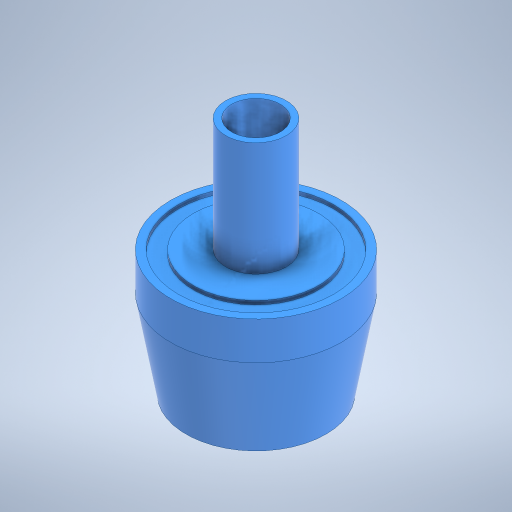
# Autodesk Inventor part: FlangeCone
Saved by Autodesk Inventor 2024 (Build 280153000, 153)
## iProperties
Created: 2023-09-22
Part Number: FlangeCone
Material: Brass
Document SubType Name: Modeling
Designer: schanen
Density: 8.49 g/cm^3
Appearance: Cyan
Author: schanen
Autodesk Inventor part; units mm, degrees
ref_plane "YZ Plane" through (0, 0, 0) normal (1, 0, 0) x (0, 1, 0)
ref_plane "XZ Plane" through (0, 0, 0) normal (0, 1, 0) x (-1, 0, 0)
ref_plane "XY Plane" through (0, 0, 0) normal (0, 0, 1) x (1, 0, 0)
sketch "Sketch1" plane through (0, 0, 0) normal (0, 0, 1) x (1, 0, 0)
  line L0 (-6.4, 63) -> (-6.4, 48)
  line L1 (-6.4, 48) -> (-6.1, 48)
  line L2 (-6.1, 48) -> (-6.1, 23)
  line L3 (-6.1, 23) -> (-17.5, 23)
  line L4 (-17.5, 23) -> (-17.5, 0)
  line L5 (-17.5, 0) -> (-18.4445, 0)
  line L6 (-18.4445, 0) -> (-22.5, 23)
  line L7 (-22.5, 23) -> (-22.5, 33)
  line L8 (-22.5, 33) -> (-20.5, 33)
  line L9 (-20.5, 33) -> (-20.5, 32)
  line L10 (-20.5, 32) -> (-16.5, 32)
  line L11 (-16.5, 32) -> (-16.5, 33)
  line L12 (-16.5, 33) -> (-8, 33)
  line L13 (-8, 33) -> (-8, 63)
  line L14 (-8, 63) -> (-6.4, 63)
  line L15 (0, -12.6) -> (0, 75.6) projected
  point P0 (0, 0)
  point P1 (-17.9722, 0)
  dimension "d0" = 23
  dimension "d1" = 15
  dimension "d2" = 30
  dimension "d3" = 10
  dimension "d4" = 17.5
  dimension "d5" = 6.1
  dimension "d6" = 6.4
  dimension "d7" = 8
  dimension "d8" = 22.5
  dimension "d9" = 10
  dimension "d10" = 4
  dimension "d11" = 20.5
  dimension "d12" = 1
  constraints: 30 end point, 11 perpendicular, 3 point on line, 1 horizontal alignment, 1 midpoint, 1 parallel, 1 vertical
  measures "d0" distance of L3.end L4.end
  measures "d1" distance of L0.start L0.end
  measures "d2" distance of L12.end L13.end
  measures "d3" distance of L6.end L7.end
  measures "d4" distance from line of point (0, 0) L4
  measures "d5" distance from line of point (0, 0) L2
  measures "d6" distance from line of point (0, 0) L0
  measures "d7" distance from line of point (0, 0) L13
  measures "d8" distance from line of point (0, 0) L7
  measures "d9" angle of L7 L6
  measures "d10" distance between parallel lines of L9 L11
  measures "d11" distance from line of point (0, 0) L9
  measures "d12" distance between parallel lines of L12 L10
revolve "Revolution1" add sketch "Sketch1" angle 360 about axis through (0, -10, 0) along (0, 1, 0)
sketch "Sketch2" plane through (0, 23, 0) normal (0, -1, 0) x (1, 0, 0)
  circle A0 centre (0, 0) radius 11 construction
  point P0 (0, 11)
  point P1 (-9.5263, -5.5)
  point P2 (9.5263, -5.5)
  dimension "d14" = 22
  dimension "d15" = 120
  dimension "d16" = 120
  constraints: 3 point on circle, 1 centre point, 1 coincident
  measures "d14" diameter of A0
hole "Hole1" at (0, 23, 11) at (-9.5263, 23, -5.5) at (9.5263, 23, -5.5) direction (0, 1, 0) diameter 2.459 depth 6 tip angle 118 thread size "M3x0.5" class "6H" standard "ANSI Metric M Profile"
body "Solid1"
